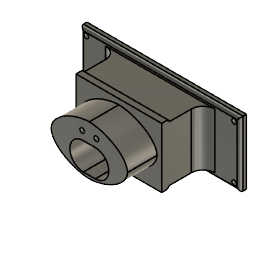
Front Camera Assembly (Autodesk Fusion 360 archive; units mm, degrees)
design "Jeep - Camera and PDB Mount"
Autodesk Fusion 360 part; units mm, degrees
sketch "Sketch1" plane through (0, 0, 0) normal (0, 1, 0) x (1, 0, 0)
  line L0 (-36.25, -23.375) -> (36.25, -23.375)
  line L1 (36.25, -23.375) -> (36.25, 23.375)
  line L2 (36.25, 23.375) -> (-36.25, 23.375)
  line L3 (-36.25, 23.375) -> (-36.25, -23.375)
  dimension "d62" = 72.5
  dimension "d63" = 46.75
  dimension "d64" = 23.375
  dimension "d65" = 36.25
  constraint horizontal L0
  constraint vertical L1
  constraint horizontal L2
  constraint vertical L3
  measures "d62" distance of L0.start L0.end
  measures "d63" distance of L0.start L2.end
  measures "d64" distance of origin L0
  measures "d65" distance of origin L3
extrude "Extrude9" add sketch "Sketch1" along normal blind 60
sketch "Sketch8" plane through (0, 0, 0) normal (0, 1, 0) x (1, 0, 0)
  line L0 (-5, -4.625) -> (5, -4.625)
  line L1 (-5, 18.375) -> (5, 18.375)
  arc A0 (-5, 18.375) -> (-5, -4.625) centre (-5, 6.875) ccw
  arc A1 (5, -4.625) -> (5, 18.375) centre (5, 6.875) ccw
  line L2 (36.25, 23.375) -> (-36.25, 23.375)
  line L3 (36.25, 23.375) -> (-36.25, 23.375)
  dimension "d39" = 10
  dimension "d40" = 5
  dimension "d94" = 23
  dimension "d123" = 28
  constraint horizontal A0.centre A1.centre
  constraint tangent L0 A1
  constraint tangent L1 A1
  constraint tangent L1 A0
  constraint tangent L0 A0
  measures "d39" distance of L0.start L0.end
  measures "d40" horizontal distance of origin A0.centre
  measures "d94" distance of L0 L1
  measures "d123" distance of L0 L3
extrude "Extrude10" cut sketch "Sketch8" along normal blind 95
sketch "Sketch9" plane through (0, 0, -23.375) normal (0, 0, -1) x (1, 0, 0)
  line L0 (36.25, 0) -> (-36.25, 0)
  line L1 (-36.25, 0) -> (-36.25, -60)
  line L2 (-36.25, -60) -> (36.25, -60)
  line L3 (36.25, -60) -> (36.25, 0)
  line L4 (-5, -33) -> (5, -33)
  line L5 (-5, -58) -> (5, -58)
  arc A0 (-5, -33) -> (-5, -58) centre (-5, -45.5) ccw
  arc A1 (5, -58) -> (5, -33) centre (5, -45.5) ccw
  dimension "d45" = 10
  dimension "d46" = 10
  dimension "d47" = 5
  dimension "d75" = 2
  dimension "d95" = 25
  constraint horizontal A0.centre A1.centre
  constraint tangent L4 A1
  constraint horizontal L4
  constraint tangent L5 A1
  constraint parallel L4 L5
  measures "d45" distance of L4.start L4.end
  measures "d46" distance of L5.start L5.end
  measures "d47" horizontal distance of origin A0.centre
  measures "d75" distance of L2 L5
  measures "d95" distance of L4 L5
extrude "Extrude11" cut sketch "Sketch9" against normal blind 12 contours L4 L5 A0 A1
sketch "Sketch10" plane through (0, 60, 0) normal (0, 1, 0) x (-1, 0, 0)
  line L0 (36.25, -23.375) -> (36.25, 23.375)
  line L1 (36.25, 23.375) -> (-36.25, 23.375)
  line L2 (-36.25, 23.375) -> (-36.25, -23.375)
  line L3 (-36.25, -23.375) -> (36.25, -23.375)
  line L4 (-67.5, 27.5) -> (67.5, 27.5)
  line L5 (67.5, 27.5) -> (67.5, -27.5)
  line L6 (67.5, -27.5) -> (-67.5, -27.5)
  line L7 (-67.5, -27.5) -> (-67.5, 27.5)
  line L8 (5, -18.375) -> (-5, -18.375)
  arc A0 (-5, 4.625) -> (-5, -18.375) centre (-5, -6.875) ccw
  line L9 (-5, 4.625) -> (5, 4.625)
  arc A1 (5, -18.375) -> (5, 4.625) centre (5, -6.875) ccw
  line L10 (57.5, -6.5) -> (57.5, -24.5)
  line L11 (57.5, -24.5) -> (-57.5, -24.5)
  line L12 (-57.5, -24.5) -> (-57.5, -1.5)
  line L13 (-57.5, -1.5) -> (-44.5, -1.5)
  line L14 (-44.5, -1.5) -> (-44.5, -6.5)
  line L15 (-57.5, -12.4536) -> (-57.5, -1.5)
  line L16 (-44.5, -6.5) -> (57.5, -6.5)
  dimension "d50" = 135
  dimension "d51" = 55
  dimension "d52" = 27.5
  dimension "d53" = 67.5
  dimension "d141" = 115
  dimension "d142" = 10
  dimension "d143" = 13
  dimension "d144" = 23
  dimension "d145" = 18
  dimension "d146" = 3
  constraint horizontal L4
  constraint vertical L5
  constraint horizontal L6
  constraint vertical L7
  constraint vertical L10
  constraint horizontal L11
  constraint vertical L12
  constraint horizontal L13
  constraint vertical L14
  constraint vertical L15
  constraint perpendicular L10 L16
  measures "d50" distance of L4.start L4.end
  measures "d51" distance of L4.start L6.end
  measures "d52" distance of origin L4
  measures "d53" distance of origin L7
  measures "d141" distance of L10.end L11.end
  measures "d142" distance of L7 L12
  measures "d143" distance of L12.end L13.end
  measures "d144" distance of L11 L13
  measures "d145" distance of L10.end L10.start
  measures "d146" distance of L6 L11
extrude "Extrude12" add sketch "Sketch10" along normal blind 5.5 contours L0 L2 L3 L8 A0 A1 L16 | L0 L2 L3 L10 L11 L12 L13 L14 L15 L16 | L0 L1 L2 A0 L9 A1 L16 | A0 L9 A1 L16 | L8 A0 A1 L16 | L4 L5 L6 L7
sketch "Sketch13" plane through (0, 0, -23.375) normal (0, 0, -1) x (1, 0, 0)
  line L0 (5, -58) -> (-5, -58)
  arc A0 (-5, -33) -> (-5, -58) centre (-5, -45.5) ccw
  line L1 (-5, -33) -> (5, -33)
  arc A1 (5, -58) -> (5, -33) centre (5, -45.5) ccw
  line L2 (36.25, 0) -> (-36.25, 0)
  line L3 (-36.25, 0) -> (-36.25, -60)
  line L4 (-36.25, -60) -> (36.25, -60)
  line L5 (36.25, -60) -> (36.25, 0)
  line L6 (-36.25, -30.2113) -> (36.25, -30.2113)
  line L7 (36.25, -30.2113) -> (36.25, -25)
  line L8 (36.25, -25) -> (-36.25, -25)
  line L9 (-36.25, -25) -> (-36.25, -30.2113)
  dimension "d113" = 25
  constraint horizontal L6
  constraint vertical L7
  constraint horizontal L8
  constraint vertical L9
  constraint coincident L5 L7.end
  constraint coincident L3 L6.start
  measures "d113" distance of L2 L8
extrude "Extrude17" add sketch "Sketch13" along normal blind 2 contours L3 L5 L6 L7 L8 L9
sketch "Sketch14" plane through (0, 65.5, 0) normal (0, 1, 0) x (-1, 0, 0)
  line L0 (-67.5, -27.5) -> (67.5, -27.5)
  line L1 (67.5, -27.5) -> (67.5, 27.5)
  line L2 (67.5, 27.5) -> (-67.5, 27.5)
  line L3 (-67.5, 27.5) -> (-67.5, -27.5)
  circle A0 centre (-62.5, 22.5) radius 2
  circle A1 centre (-62.5, -22.5) radius 2
  circle A2 centre (62.5, 22.5) radius 2
  circle A3 centre (62.5, -22.5) radius 2
  dimension "d78" = 4
  dimension "d79" = 4
  dimension "d80" = 4
  dimension "d81" = 4
  dimension "d83" = 5
  dimension "d84" = 5
  dimension "d85" = 5
  dimension "d86" = 5
  dimension "d88" = 5
  dimension "d89" = 5
  dimension "d90" = 5
  dimension "d91" = 5
  measures "d78" diameter of A0
  measures "d79" diameter of A2
  measures "d80" diameter of A3
  measures "d81" diameter of A1
  measures "d83" distance of L1 A3.centre
  measures "d84" distance of L1 A2.centre
  measures "d85" distance of L3 A0.centre
  measures "d86" distance of L3 A1.centre
  measures "d88" distance of L2 A0.centre
  measures "d89" distance of L2 A2.centre
  measures "d90" distance of L0 A3.centre
  measures "d91" distance of L0 A1.centre
extrude "Extrude18" cut sketch "Sketch14" against normal blind 15 contours A0 | A1 | A2 | A3
fillet "Fillet1" radius 2 2 edges at (0, 30.2113, -25.375) (0, 30.2113, -23.375)
sketch "Sketch15" plane through (0, 0, 0) normal (0, -1, 0) x (1, 0, 0)
  line L0 (5, -18.375) -> (-5, -18.375)
  arc A0 (-5, 4.625) -> (-5, -18.375) centre (-5, -6.875) ccw
  line L1 (-5, 4.625) -> (5, 4.625)
  arc A1 (5, -18.375) -> (5, 4.625) centre (5, -6.875) ccw
  line L2 (-36.25, 23.375) -> (-36.25, -23.375)
  line L3 (-36.25, -23.375) -> (36.25, -23.375)
  line L4 (36.25, -23.375) -> (36.25, 23.375)
  line L5 (36.25, 23.375) -> (-36.25, 23.375)
  circle A2 centre (-6, 11.5) radius 2
  circle A3 centre (6, 11.5) radius 2
  dimension "d99" = 4
  dimension "d100" = 4
  dimension "d101" = 12
  dimension "d102" = 6
  dimension "d103" = 6
  dimension "d140" = 11.5
  constraint horizontal A2.centre A3.centre
  measures "d99" diameter of A3
  measures "d100" diameter of A2
  measures "d101" distance of A2.centre A3.centre
  measures "d102" horizontal distance of origin A2.centre
  measures "d103" horizontal distance of origin A3.centre
  measures "d140" vertical distance of origin A2.centre
extrude "Extrude19" cut sketch "Sketch15" against normal blind 20 contours A2 | A3
ref_plane "WorkPlane1" through (0, 30, 0) normal (0, 0, -1) x (-1, 0, 0)
mirror "Mirror2" about plane through (0, 30, 0) normal (0, 0, -1) of "Extrude17"
sketch "Sketch17" plane through (0, 0, 0) normal (0, -1, 0) x (1, 0, 0)
  line L0 (5, -18.375) -> (-5, -18.375)
  arc A0 (-5, 4.625) -> (-5, -18.375) centre (-5, -6.875) ccw
  line L1 (-5, 4.625) -> (5, 4.625)
  arc A1 (5, -18.375) -> (5, 4.625) centre (5, -6.875) ccw
  line L2 (-36.25, 23.375) -> (-36.25, -23.375)
  line L3 (-36.25, -23.375) -> (36.25, -23.375)
  line L4 (36.25, -23.375) -> (36.25, 23.375)
  line L5 (36.25, 23.375) -> (-36.25, 23.375)
  circle A2 centre (-5, -6.875) radius 3
  circle A3 centre (5, -6.875) radius 3
  line L6 (-5, 4.625) -> (5, 4.625)
  line L7 (-5, -18.375) -> (5, -18.375)
  circle A4 centre (-6, 11.5) radius 2
  circle A5 centre (6, 11.5) radius 2
  dimension "d114" = 6
  constraint concentric A0 A2
  constraint concentric A1 A3
  constraint coincident A0.start L1.start
  constraint coincident L1.end A1.end
  constraint coincident L0.end A0.end
  constraint coincident L0.start A1.start
  measures "d114" diameter of A3
fillet "Fillet3" radius 2.5 4 edges at (0, 60, 27.5) (-67.5, 60, 0) (67.5, 60, 0) (0, 60, -27.5)
fillet "Fillet7" radius 2 1 edges at (0, 30.2113, 23.375)
fillet "Fillet10" radius 10 2 edges at (36.25, 60, 0) (-36.25, 60, 0)
sketch "Sketch18" plane through (0, 0, 0) normal (0, -1, 0) x (1, 0, 0)
  circle A0 centre (-6, 11.5) radius 2
  circle A1 centre (6, 11.5) radius 2
  line L0 (5, -18.375) -> (-5, -18.375)
  arc A2 (-5, 4.625) -> (-5, -18.375) centre (-5, -6.875) ccw
  line L1 (-5, 4.625) -> (5, 4.625)
  arc A3 (5, -18.375) -> (5, 4.625) centre (5, -6.875) ccw
  line L2 (-36.25, 23.375) -> (-36.25, -23.375)
  line L3 (-36.25, -23.375) -> (36.25, -23.375)
  line L4 (36.25, -23.375) -> (36.25, 23.375)
  line L5 (36.25, 23.375) -> (-36.25, 23.375)
  line L6 (-33.75, -20.875) -> (33.75, -20.875)
  line L7 (33.75, -20.875) -> (33.75, 20.875)
  line L8 (33.75, 20.875) -> (-33.75, 20.875)
  line L9 (-33.75, 20.875) -> (-33.75, -20.875)
  dimension "d134" = -2.5
extrude "Extrude21" cut sketch "Sketch18" against normal blind 25 contours L2 L3 L4 L5
sketch "Sketch19" plane through (0, 0, 0) normal (0, -1, 0) x (1, 0, 0)
  line L0 (33.75, 20.875) -> (-33.75, 20.875)
  line L1 (-33.75, 20.875) -> (-33.75, -20.875)
  line L2 (-33.75, -20.875) -> (33.75, -20.875)
  line L3 (33.75, -20.875) -> (33.75, 20.875)
  circle A0 centre (-6, 11.5) radius 2
  circle A1 centre (6, 11.5) radius 2
  line L4 (5, -18.375) -> (-5, -18.375)
  arc A2 (-5, 4.625) -> (-5, -18.375) centre (-5, -6.875) ccw
  line L5 (-5, 4.625) -> (5, 4.625)
  arc A3 (5, -18.375) -> (5, 4.625) centre (5, -6.875) ccw
  line L6 (-32.4071, 0) -> (-31.9234, 9.9156) construction
  line L7 (-31.9234, 9.9156) -> (-18.8638, 18.622) construction
  line L8 (-18.8638, 18.622) -> (-5.8043, 20.875) construction
  line L9 (-5.8043, 20.875) -> (0, 20.875) construction
  spline S0 degree 4 poles (-32.4071, 0) (-31.9234, 9.9156) (-18.8638, 18.622) (-5.8043, 20.875) (0, 20.875) knots 0 0 0 0 0 1 1 1 1 1
  line L10 (-78.035, 0) -> (72.5532, 0) construction
  line L11 (0, 0) -> (0, 55.866) construction
  spline S1 degree 4 poles (32.4071, 0) (31.9234, 9.9156) (18.8638, 18.622) (5.8043, 20.875) (0, 20.875) knots 0 0 0 0 0 1 1 1 1 1
  line L12 (32.4071, 0) -> (31.9234, 9.9156) construction
  line L13 (31.9234, 9.9156) -> (18.8638, 18.622) construction
  line L14 (18.8638, 18.622) -> (5.8043, 20.875) construction
  line L15 (5.8043, 20.875) -> (0, 20.875) construction
  spline S2 degree 4 poles (-32.4071, 0) (-31.9234, -9.9156) (-18.8638, -18.622) (-5.8043, -20.875) (0, -20.875) knots 0 0 0 0 0 1 1 1 1 1
  line L16 (-32.4071, 0) -> (-31.9234, -9.9156) construction
  line L17 (-31.9234, -9.9156) -> (-18.8638, -18.622) construction
  line L18 (-18.8638, -18.622) -> (-5.8043, -20.875) construction
  line L19 (-5.8043, -20.875) -> (0, -20.875) construction
  spline S3 degree 4 poles (32.4071, 0) (31.9234, -9.9156) (18.8638, -18.622) (5.8043, -20.875) (0, -20.875) knots 0 0 0 0 0 1 1 1 1 1
  line L20 (32.4071, 0) -> (31.9234, -9.9156) construction
  line L21 (31.9234, -9.9156) -> (18.8638, -18.622) construction
  line L22 (18.8638, -18.622) -> (5.8043, -20.875) construction
  line L23 (5.8043, -20.875) -> (0, -20.875) construction
  constraint midpoint L0 L9.end
  constraint coincident L0 L8.end
  constraint perpendicular L1 L10
  constraint coincident L11.start origin
  constraint perpendicular L10 L11
  constraint symmetric L6.start L11 S1.start
  constraint symmetric L9.end L11 S0.end
  constraint symmetric S0 L11 S1
  constraint symmetric L6.start L10 S0.start
  constraint symmetric L9.end L10 S2.end
  constraint symmetric S0 L10 S2
  constraint symmetric L10 S1.start L12.start
  constraint symmetric L10 L9.end S2.end
  constraint symmetric L10 S1 S3
extrude "Extrude22" cut sketch "Sketch19" against normal blind 25 contours L0 L2 L3 S1 S3 | L0 L1 L2 S0 S2
sketch "Sketch20" plane through (0, 65.5, 0) normal (0, 1, 0) x (-1, 0, 0)
  line L0 (-44.5, -6.5) -> (57.5, -6.5)
  line L1 (-44.5, -1.5) -> (-44.5, -6.5)
  line L2 (-57.5, -1.5) -> (-44.5, -1.5)
  line L3 (57.5, -6.5) -> (57.5, -24.5)
  line L4 (-57.5, -24.5) -> (-57.5, -1.5)
  line L5 (57.5, -24.5) -> (-57.5, -24.5)
  line L6 (-57.5, -12.4536) -> (-57.5, -1.5)
  line L7 (-67.5, -27.5) -> (-67.5, 27.5)
  line L8 (67.5, -27.5) -> (-67.5, -27.5)
  dimension "d147" = 115
  dimension "d148" = 13
  dimension "d149" = 23
  dimension "d150" = 18
  dimension "d151" = 10
  dimension "d152" = 3
  constraint vertical L3
  constraint horizontal L5
  constraint vertical L4
  constraint horizontal L2
  constraint vertical L1
  constraint vertical L6
  constraint perpendicular L0 L3
  measures "d147" distance of L3.end L4.start
  measures "d148" distance of L1.start L2.start
  measures "d149" distance of L2 L5
  measures "d150" distance of L0.end L3.end
  measures "d151" distance of L4 L7
  measures "d152" distance of L5 L8
extrude "Extrude23" cut sketch "Sketch20" against normal blind 3.5
equation "d52 = ( 55 / 2 ) * 1 mm"
equation "d53 = ( 135 / 2 ) * 1 mm"
equation "d64 = ( 46.75 / 2 ) * 1 mm"
equation "d65 = ( 72.5 / 2 ) * 1 mm"
equation "d108 = -( ( 46.75 / 2 ) * 1 mm )"
